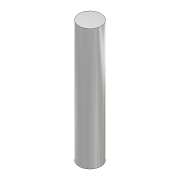
# Autodesk Inventor part: Part3
Saved by Autodesk Inventor 2017 (Build 210142000, 142)
## iProperties
Created: 2023-11-15
Part Number: Part3
Material: Generic
Document SubType Name: Modeling
Designer: Ok
Density: 1 g/cm^3
Appearance: Default
Author: Ok
Autodesk Inventor part; units mm, degrees
ref_plane "YZ Plane" through (0, 0, 0) normal (1, 0, 0) x (0, 1, 0)
ref_plane "XY Plane" through (0, 0, 0) normal (0, 0, 1) x (1, 0, 0)
sketch "Sketch1" plane through (0, 0, 0) normal (0, 0, 1) x (1, 0, 0)
  circle A0 centre (0, 0) radius 4.5
  dimension "d0" = 9
  constraints: 1 centre point, 1 coincident
  measures "d0" diameter of A0
extrude "Extrusion1" add sketch "Sketch1" along normal mid plane 50
ref_plane "Work Plane1" through (0, 4.5, 0) normal (0, 1, 0) x (-1, 0, 0)
sketch "Sketch2" plane through (0, 4.5, 0) normal (0, 1, 0) x (-1, 0, 0)
  circle A0 centre (0, -10.5) radius 2
  line L0 (-4.5, -25) -> (4.5, -25) projected
  point P0 (0, 0)
  dimension "d4" = 4
  dimension "d5" = 14.5
  constraints: 1 centre point
  measures "d4" diameter of A0
  measures "d5" distance from line of L0 A0.centre
extrude "Extrusion2" cut sketch "Sketch2" against normal blind 6
body "Solid1"
